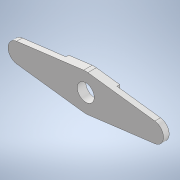
# Autodesk Inventor part: NyArm
Saved by Autodesk Inventor 2022 (Build 260153000, 153)
## iProperties
Created: 2022-06-06
Part Number: NyArm
Material: Generic
Document SubType Name: Modeling
Designer: frede
Density: 1 g/cm^3
Appearance: Default
Author: frede
Autodesk Inventor part; units mm, degrees
ref_plane "YZ Plane" through (0, 0, 0) normal (1, 0, 0) x (0, 1, 0)
ref_plane "XZ Plane" through (0, 0, 0) normal (0, 1, 0) x (-1, 0, 0)
ref_plane "XY Plane" through (0, 0, 0) normal (0, 0, 1) x (1, 0, 0)
sketch "Sketch1" plane through (0, 0, 0) normal (0, 0, 1) x (1, 0, 0)
  line L0 (24.4369, 3.4726) -> (0.749, 6.4531)
  arc A0 (0.749, 6.4531) -> (-0.749, 6.4531) centre (0, 0.5) ccw
  line L1 (-0.749, 6.4531) -> (-24.4369, 3.4726)
  arc A1 (-24.4369, 3.4726) -> (-24.4369, -3.4726) centre (-24, 0) ccw
  line L2 (-24.4369, -3.4726) -> (-0.749, -6.4531)
  arc A2 (-0.749, -6.4531) -> (0.749, -6.4531) centre (0, -0.5) ccw
  line L3 (0.749, -6.4531) -> (24.4369, -3.4726)
  arc A3 (24.4369, -3.4726) -> (24.4369, 3.4726) centre (24, 0) ccw
  circle A4 centre (0, 0) radius 3
  dimension "d0" = 55
  dimension "d1" = 13
  dimension "d2" = 6
  dimension "d3" = 3.5
  dimension "d4" = 6
  constraints: 8 end point, 8 point on circle, 8 tangent, 5 centre point, 3 equal length, 2 equal radius, 2 horizontal alignment, 2 vertical alignment, 1 coincident
  measures "d2" diameter of A4
  measures "d3" radius of A3
  measures "d4" radius of A0
extrude "Extrusion1" add sketch "Sketch1" along normal blind 2
sketch "Sketch2" plane through (0, 0, 0) normal (0, 0, -1) x (-1, 0, 0)
  arc A0 (0.749, 6.4531) -> (-0.749, 6.4531) centre (0, 0.5) ccw projected
  line L0 (-24.4369, 3.4726) -> (-0.749, 6.4531) projected
  arc A1 (-24.4369, 3.4726) -> (-24.4369, -3.4726) centre (-24, 0) ccw construction
  line L1 (-0.749, -6.4531) -> (-24.4369, -3.4726) projected
  arc A2 (-0.749, -6.4531) -> (0.749, -6.4531) centre (0, -0.5) ccw projected
  line L2 (24.4369, -3.4726) -> (0.749, -6.4531) projected
  arc A3 (24.4369, -3.4726) -> (24.4369, 3.4726) centre (24, 0) ccw construction
  line L3 (0.749, 6.4531) -> (24.4369, 3.4726) projected
  circle A4 centre (0, 0) radius 3 projected
  line L4 (-9, 5.4149) -> (-9, -5.4149)
  line L5 (-24.4369, 3.4726) -> (-0.749, 6.4531) construction
  line L6 (9, 5.4149) -> (9, -5.4149)
  line L7 (0.749, 6.4531) -> (24.4369, 3.4726) construction
  dimension "d7" = 18
  dimension "d8" = 9
  constraints: 4 end point, 4 point on line, 2 vertical
  measures "d7" distance between parallel lines of L6 L4
  measures "d8" distance from line of point (0, 0) L4
extrude "Extrusion2" add sketch "Sketch2" along normal blind 1
body "Solid1"
